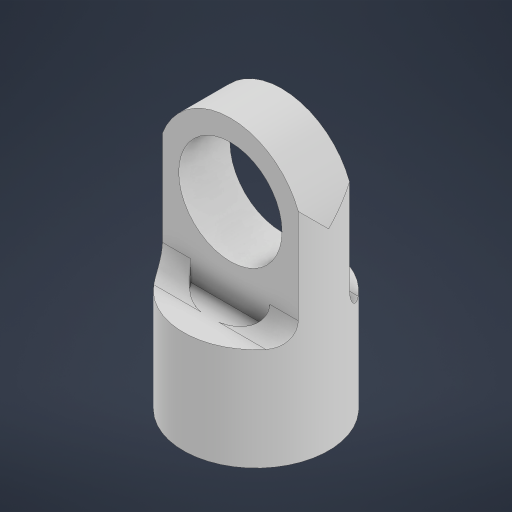
# Autodesk Inventor part: Clip
Saved by Autodesk Inventor 2024 (Build 280153000, 153)
## iProperties
Created: 2025-09-10
Part Number: Clip
Material: Generic
Document SubType Name: Modeling
Designer: kevin
Density: 1 g/cm^3
Appearance: Default
Author: kevin
Autodesk Inventor part; units mm, degrees
ref_plane "YZ Plane" through (0, 0, 0) normal (1, 0, 0) x (0, 1, 0)
ref_plane "XZ Plane" through (0, 0, 0) normal (0, 1, 0) x (-1, 0, 0)
ref_plane "XY Plane" through (0, 0, 0) normal (0, 0, 1) x (1, 0, 0)
sketch "Sketch1" plane through (0, 0, 0) normal (0, 1, 0) x (-1, 0, 0)
  circle A0 centre (0, 0) radius 8.5
  circle A1 centre (0, 0) radius 5.5
  dimension "d0" = 17
  dimension "d1" = 11
  constraints: 2 centre point, 2 coincident
  measures "d0" diameter of A0
  measures "d1" diameter of A1
extrude "Extrusion1" add sketch "Sketch1" along normal blind 12
sketch "Sketch3" plane through (0, 0, 0) normal (0, 0, 1) x (1, 0, 0)
  line L0 (8.5, 12) -> (-8.5, 12) projected
  line L1 (8.5, 0) -> (-8.5, 0) projected
  circle A0 centre (0, 22.4852) radius 8.5
  line L2 (-8.5, 22.4852) -> (-8.5, 12)
  line L3 (8.5, 22.4852) -> (8.5, 12)
  circle A1 centre (0, 22.4852) radius 6.05
  point P0 (0, 0)
  dimension "d4" = 17
  dimension "d5" = 12.1
  constraints: 4 end point, 2 centre point, 2 point on circle, 2 vertical, 1 coincident
  measures "d4" diameter of A0
  measures "d5" diameter of A1
extrude "Extrusion2" add sketch "Sketch3" along normal mid plane 6
sketch "Sketch4" plane through (-4.6098, 12, 3) normal (0, -1, 0) x (1, 0, 0)
  circle A0 centre (4.6098, -3) radius 5.5 projected
  arc A1 (13.1098, -3) -> (12.5628, 0) centre (4.6098, -3) ccw projected
  line L0 (13.1098, -3) -> (13.1098, 0) projected
  line L1 (12.5628, 0) -> (13.1098, 0) projected
  arc A2 (12.5628, -6) -> (13.1098, -3) centre (4.6098, -3) ccw projected
  line L2 (13.1098, -6) -> (12.5628, -6) projected
  line L3 (13.1098, -6) -> (13.1098, -3) projected
  arc A3 (-3.3432, 0) -> (-3.8902, -3) centre (4.6098, -3) ccw projected
  line L4 (-3.8902, 0) -> (-3.3432, 0) projected
  line L5 (-3.8902, -3) -> (-3.8902, 0) projected
  arc A4 (-3.8902, -3) -> (-3.3432, -6) centre (4.6098, -3) ccw projected
  line L6 (-3.8902, -6) -> (-3.8902, -3) projected
  line L7 (-3.3432, -6) -> (-3.8902, -6) projected
  point P0 (-3.8902, -3)
  point P1 (-3.8902, -3)
  point P2 (-3.8902, -3)
  point P3 (-3.8902, -3)
extrude "Extrusion4" cut sketch "Sketch4" against normal blind 37.425 contours A1 L1 L0 | L3 L2 A2 | A4 L7 L6 | A3 L5 L4
fillet "Fillet1" radius 2.4 4 edges at (6.2814, 12, -3) (-6.2814, 12, -3) (-6.2814, 12, 3) (6.2814, 12, 3)
extrude "Extrusion5" add sketch "Sketch4" along normal blind 2.5 contours A0
body "Solid1"
